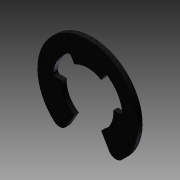
# Autodesk Inventor part: e-clip
Saved by Autodesk Inventor 2012 (Build 160160000, 160)
## iProperties
Created: 2009-01-30
Part Number: e-clip
Material: Steel, Mild
Document SubType Name: Modeling
Designer: Administrator
Density: 7.86 g/cm^3
Author: Administrator
Autodesk Inventor part; units mm, degrees
ref_plane "YZ Plane" through (0, 0, 0) normal (1, 0, 0) x (0, 1, 0)
ref_plane "XZ Plane" through (0, 0, 0) normal (0, 1, 0) x (-1, 0, 0)
ref_plane "XY Plane" through (0, 0, 0) normal (0, 0, 1) x (1, 0, 0)
sketch "Sketch1" plane through (0, 0, 0) normal (0, 0, 1) x (1, 0, 0)
  line L0 (-14.6304, 0) -> (19.5072, 0) projected
  line L1 (0, -14.6304) -> (0, 19.5072) projected
  circle A0 centre (0, 0) radius 6.096 construction
  circle A1 centre (0, 0) radius 12.192 construction
  arc A2 (7.9579, -8.8987) -> (-7.9579, -8.8987) centre (0, 0) ccw
  arc A3 (3.175, 5.2039) -> (-3.175, 5.2039) centre (0, 0) ccw
  arc A4 (-6.0799, 0.4427) -> (-3.175, -5.2039) centre (0, 0) ccw
  arc A5 (3.175, -5.2039) -> (6.0799, 0.4427) centre (0, 0) ccw
  circle A6 centre (0, 0) radius 8.255 construction
  arc A7 (-4.8834, 6.6557) -> (-8.1645, 1.219) centre (0, 0) ccw
  arc A8 (8.1645, 1.219) -> (4.8834, 6.6557) centre (0, 0) ccw
  line L2 (-3.175, 5.2039) -> (-3.937, 6.5237)
  line L3 (3.175, 5.2039) -> (3.937, 6.5237)
  line L4 (6.0799, 0.4427) -> (7.6039, 0.4427)
  line L5 (-6.0799, 0.4427) -> (-7.6039, 0.4427)
  line L6 (-3.175, -5.2039) -> (-5.0383, -8.4312)
  line L7 (3.175, -5.2039) -> (5.0383, -8.4312)
  arc A9 (-8.1645, 1.219) -> (-7.6039, 0.4427) centre (-7.4868, 1.1178) ccw
  arc A10 (-3.937, 6.5237) -> (-4.8834, 6.6557) centre (-4.478, 6.1032) ccw
  arc A11 (4.8834, 6.6557) -> (3.937, 6.5237) centre (4.478, 6.1032) ccw
  arc A12 (7.6039, 0.4427) -> (8.1645, 1.219) centre (7.4868, 1.1178) ccw
  arc A13 (-7.9579, -8.8987) -> (-5.0383, -8.4312) centre (-6.6881, -7.4787) ccw
  arc A14 (5.0383, -8.4312) -> (7.9579, -8.8987) centre (6.6881, -7.4787) ccw
  point P0 (0, 6.096)
  dimension "d0" = 12.192
  dimension "d1" = 24.384
  dimension "d2" = 23.876
  dimension "d4" = 6.35
  dimension "d5" = 6.35
  dimension "d6" = 6.35
  dimension "d7" = 16.51
  dimension "d9" = 30
  dimension "d13" = 1.524
  dimension "d14" = 6.35
  dimension "d15" = 6.35
  dimension "d16" = 60
  dimension "d17" = 60
  dimension "d18" = 30
  dimension "d19" = 1.905
  constraints: 35 point on circle, 15 centre point, 12 end point, 8 tangent, 7 equal radius, 4 coincident, 3 equal length, 3 vertical alignment, 1 concentric, 1 horizontal alignment, 2 other
  measures "d0" diameter of A0
  measures "d1" diameter of A1
  measures "d2" diameter of A2
  measures "d4" distance of L3.start L2.start
  measures "d5" distance of L6.start L5.start
  measures "d6" distance of L7.start L4.start
  measures "d7" diameter of A6
  measures "d9" angle of L1 L2
  measures "d13" distance of L4.start L4.end
  measures "d14" distance of A6.end A6.start
  measures "d15" distance of A8.start A8.end
  measures "d16" angle of L2 L5
  measures "d17" angle of L4 L3
  measures "d18" angle of L1 L7
  measures "d19" radius of A13
extrude "Extrusion1" add sketch "Sketch1" along normal mid plane 1.0668 contours A2 L1 A3 L2 A10 A7 A9 L5 A4 L0 | L0 A4 L6 A13 A2 | A2 L0 A5 L4 A12 A8 A11 L3 A3 L1 | A2 A14 L7 A5 L0
body "Solid1"
